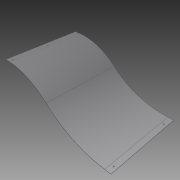
# Autodesk Inventor part: Bounce Polycarbonate Flap
Saved by Autodesk Inventor 2014 SP1 (Build 180222100, 222)
## iProperties
Created: 2013-12-17
Part Number: Bounce Polycarbonate Flap
Material: Polycarbonate, Clear
Document SubType Name: Modeling
Designer: Moses
Mass: 72.5357 g
Surface Area: 1532.48 cm^2
Volume: 60.4464 cm^3
Density: 1.2 g/cm^3
Appearance: Polycarbonate - Clear
Author: Moses
Autodesk Inventor part; units mm, degrees
ref_plane "YZ Plane" through (0, 0, 0) normal (1, 0, 0) x (0, 1, 0)
ref_plane "XZ Plane" through (0, 0, 0) normal (0, 1, 0) x (-1, 0, 0)
ref_plane "Work Plane1" through (0, 0, 0) normal (0, 0, 1) x (1, 0, 0)
sketch "Sketch1" plane through (0, 0, 0) normal (0, 0, 1) x (1, 0, 0)
  line L0 (165.1, 107.5162) -> (-165.1, 107.5162) construction
  line L1 (-165.1, 107.5162) -> (-165.1, 110.6912) construction
  line L2 (165.1, 110.6912) -> (-165.1, 110.6912) construction
  line L3 (165.1, 107.5162) -> (165.1, 110.6912) construction
  line L4 (161.925, -1.2275) -> (161.925, 14.6475) construction
  line L5 (161.925, 14.6475) -> (161.1313, 14.6475) construction
  line L6 (161.1313, 14.6475) -> (161.1313, -0.4338) construction
  line L7 (161.1313, -0.4338) -> (146.05, -0.4338) construction
  line L8 (146.05, -0.4338) -> (146.05, -1.2275) construction
  line L9 (146.05, -1.2275) -> (161.925, -1.2275) construction
  line L10 (-153.9875, 110.6912) -> (-150.8125, 110.6912) construction
  line L11 (161.925, -1.2275) -> (146.05, -1.2275)
  arc A0 (-23.8125, 60.9948) -> (-150.8125, 107.5162) centre (-150.8125, -89.0948) ccw
  arc A1 (-23.8125, 60.9948) -> (146.05, -1.2275) centre (146.05, 261.7398) ccw
  line L12 (-150.8125, 110.6912) -> (-150.8125, 107.5162) construction
  line L13 (-150.8125, 107.5162) -> (-165.1, 107.5162)
  arc A2 (-24.3252, 60.3889) -> (-150.8125, 106.7225) centre (-150.8125, -89.0948) ccw
  arc A3 (-24.3252, 60.3889) -> (146.05, -2.0213) centre (146.05, 261.7398) ccw
  line L14 (146.05, -2.0213) -> (161.925, -2.0213)
  line L15 (-165.1, 107.5162) -> (-165.1, 106.7225)
  line L16 (-165.1, 106.7225) -> (-150.8125, 106.7225)
  line L17 (161.925, -1.2275) -> (161.925, -2.0213)
  point P0 (0, 0)
  dimension "d8" = 127
  dimension "d9" = 0.7937
  constraints: 14 end point, 8 point on circle, 4 centre point, 4 tangent, 3 horizontal, 3 vertical, 1 point on line, 2 other
  measures "d8" horizontal distance of L12.end A0.start
  measures "d9" distance of L12.end L16.end
extrude "Extrusion1" add sketch "Sketch1" along normal blind 215.9
sketch "Sketch2" plane through (-165.1, 106.7225, 0) normal (0, -1, 0) x (1, 0, 0)
  circle A0 centre (12.7, 3.175) radius 1.5875
  circle A1 centre (12.7, 104.775) radius 1.5875
  circle A2 centre (12.7, 206.375) radius 1.5875
  line L0 (14.2875, 0) -> (0, 0) projected
  line L1 (14.2875, 0) -> (14.2875, 215.9) projected
  line L2 (0, 215.9) -> (14.2875, 215.9) projected
  line L3 (0, 0) -> (0, 215.9) projected
  point P0 (165.1, 0)
  constraints: 3 centre point
extrude "Extrusion2" cut sketch "Sketch2" against normal through all contours A0 | A1 | A2
sketch "Sketch3" plane through (146.05, -1.2275, 0) normal (0, 1, 0) x (1, 0, 0)
  circle A0 centre (7.5406, -198.5968) radius 1.5875 projected
  circle A1 centre (7.5406, -27.1468) radius 1.5875 projected
  point P0 (-146.05, 0)
extrude "Extrusion3" cut sketch "Sketch3" against normal through all
body "Solid1"
